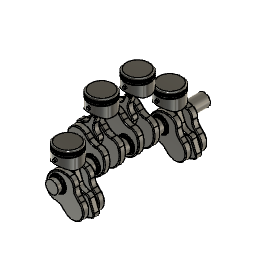
piston sim (v6~recovered) (Autodesk Fusion 360 design; units mm, degrees)
Autodesk Fusion 360 part; units mm, degrees
note: some values were not read from the file. Set by a fixed rule: which face or edge a step refers to.
sketch "Sketch1" plane through (0, 0, 0) normal (0, 1, 0) x (1, 0, 0) in component "piston2"
  line L0 (0, 0) -> (40, 0)
  line L1 (40, 0) -> (40, -55)
  line L2 (40, -55) -> (0, -55)
  line L3 (0, -55) -> (0, 0)
  line L4 (40, -48) -> (36, -48)
  line L5 (36, -48) -> (36, -46)
  line L6 (36, -46) -> (40, -46)
  line L7 (40, -46) -> (40, -48)
  line L8 (40, -44) -> (36, -44)
  line L9 (36, -44) -> (36, -42)
  line L10 (36, -42) -> (40, -42)
  line L11 (40, -42) -> (40, -44)
  line L12 (40, -38) -> (36, -38)
  line L13 (36, -38) -> (36, -36)
  line L14 (36, -36) -> (40, -36)
  line L15 (40, -36) -> (40, -38)
  dimension "d1" = 40
  dimension "d2" = 55
  dimension "d3" = 2
  dimension "d4" = 7
  dimension "d5" = 4
  dimension "d6" = 4
  dimension "d7" = 2
  dimension "d8" = 2
  dimension "d9" = 4
  dimension "d10" = 2
  dimension "d11" = 4
  constraint horizontal L0
  constraint vertical L1
  constraint horizontal L2
  constraint vertical L3
  constraint coincident L0.start L3.end
  constraint horizontal L4
  constraint vertical L5
  constraint horizontal L6
  constraint vertical L7
  constraint coincident L1 L4.start
  constraint horizontal L8
  constraint vertical L9
  constraint horizontal L10
  constraint vertical L11
  constraint coincident L1 L8.start
  constraint horizontal L12
  constraint vertical L13
  constraint horizontal L14
  constraint vertical L15
  constraint coincident L1 L12.start
  measures "d1" distance of L0.start L0.end
  measures "d2" distance of L0.start L2.end
  measures "d3" distance of L4.end L5.end
  measures "d4" distance of L1.end L4.start
  measures "d5" distance of L4.start L4.end
  measures "d6" distance of L8.start L8.end
  measures "d7" distance of L8.end L9.end
  measures "d8" distance of L12.end L13.end
  measures "d9" distance of L12.start L12.end
  measures "d10" distance of L6.end L8.start
  measures "d11" distance of L10.end L12.start
revolve "Revolve1" add sketch "Sketch1" angle 360 about axis through (0, 0, 55) along (0, 0, -1) contours L0 L1 L2 L3 L4 L5 L6 L8 L9 L10 L12 L13 L14 makes body 1 in component "piston2"
fillet "Fillet1" radius 5 1 edges at (-37.2931, -14.4646, 55) on bodies 1 in component "piston2"
sketch "Sketch2" plane through (0, 0, 0) normal (0, 0, -1) x (1, 0, 0) in component "piston2"
  circle A0 centre (0, 0) radius 40
  circle A1 centre (0, 0) radius 35
  dimension "d15" = 70
  constraint coincident A0.centre A1.centre
  measures "d15" diameter of A1
extrude "Extrude1" cut sketch "Sketch2" against normal blind 50 contours A1 bodies 1 in component "piston2"
sketch "Sketch3" plane through (0, 0, 0) normal (0, 1, 0) x (1, 0, 0) in component "piston2"
  line L0 (-40, 0) -> (40, 0)
  line L1 (-40, -36) -> (40, -36)
  line L2 (0, 0) -> (0, -10)
  circle A0 centre (0, -24) radius 5
  arc A1 (-35, 0) -> (35.5, 0) centre (0.25, 56.0937) ccw
  point P0 (-35, 0)
  dimension "d18" = 10
  dimension "d19" = 10
  dimension "d22" = 5
  dimension "d23" = 4.5
  dimension "d24" = 5
  dimension "d25" = 24
  constraint coincident L2.start origin
  constraint perpendicular L0 L2
  constraint coincident L0 A1.end
  constraint coincident P0 A1.start
  measures "d18" distance of L2.start L2.end
  measures "d19" diameter of A0
  measures "d22" distance of L0.start P0
  measures "d23" distance of L0.end A1.end
  measures "d24" distance of L0.start P0
  measures "d25" distance of L2.start A0.centre
extrude "Extrude2" cut sketch "Sketch3" along normal blind 45 and the other way blind 55 bodies 1 in component "piston2"
pattern_linear "00000000-0000-0000-0000-000000000000" [suppressed] in component "pistons"
sketch "Sketch1 (2)" plane through (0, 0, 0) normal (0, 1, 0) x (1, 0, 0) in component "connecting rod"
  circle A0 centre (0, -75) radius 5
  circle A1 centre (0, -75) radius 8.5
  circle A2 centre (0, 50) radius 22.5
  line L0 (8.5, -75) -> (8.5, 0)
  line L1 (0, 50) -> (36, 50)
  line L2 (36, 50) -> (36, 25)
  line L3 (36, 25) -> (33.5, 25)
  arc A3 (33.5, 25) -> (8.5, 0) centre (33.5, 0) ccw
  line L4 (0, 0) -> (0, 50) construction
  line L5 (-8.5, -75) -> (-8.5, 0)
  arc A4 (-8.5, 0) -> (-33.5, 25) centre (-33.5, 0) ccw
  line L6 (-36, 50) -> (-36, 25)
  line L7 (-36, 25) -> (-33.5, 25)
  line L8 (0, 50) -> (-36, 50)
  line L9 (-36, 50) -> (36, 50)
  line L10 (36, 50) -> (36, 86)
  line L11 (36, 86) -> (-36, 86)
  line L12 (-36, 86) -> (-36, 50)
  circle A5 centre (0, -60) radius 4.75
  circle A6 centre (0, -23) radius 4.75
  line L13 (-4.75, -60) -> (-4.75, -23)
  line L14 (4.75, -60) -> (4.75, -23)
  dimension "d34" = 10
  dimension "d35" = 17
  dimension "d36" = 45
  dimension "d37" = 125
  dimension "d39" = 36
  dimension "d40" = 25
  dimension "d41" = 25
  dimension "d42" = 36
  dimension "d47" = 9.5
  dimension "d48" = 15
  dimension "d49" = 15
  dimension "d60" = 37
  dimension "d61" = 9.5
  constraint concentric A0 A1
  constraint coincident A1 L0.start
  constraint tangent A1 L0
  constraint vertical L0
  constraint coincident A2.centre L1.start
  constraint horizontal L1
  constraint perpendicular L1 L2
  constraint perpendicular L0 L3
  constraint tangent L3 A3
  constraint tangent L0 A3
  constraint coincident L4.start origin
  constraint perpendicular L1 L4
  constraint symmetric L0.start L4 L5.start
  constraint symmetric A2.centre L4 L1.start
  constraint symmetric L1.end L4 L6.start
  constraint symmetric L2.end L4 L6.end
  constraint symmetric L3.end L4 A4.end
  constraint symmetric L0.end L4 L5.end
  constraint symmetric A3 L4 A4
  constraint horizontal L9
  constraint vertical L10
  constraint horizontal L11
  constraint vertical L12
  constraint coincident A5 L13.start
  constraint tangent A5 L13
  constraint coincident A6 L13.end
  constraint tangent A6 L13
  constraint vertical L13
  constraint coincident A5 L14.start
  constraint tangent A5 L14
  constraint coincident A6 L14.end
  constraint tangent A6 L14
  measures "d34" diameter of A0
  measures "d35" diameter of A1
  measures "d36" diameter of A2
  measures "d37" distance of A0.centre A2.centre
  measures "d39" distance of A2.centre L1.end
  measures "d40" distance of L1.end L2.end
  measures "d41" radius of A3
  measures "d42" distance of L6.start L11.end
  measures "d47" diameter of A5
  measures "d48" distance of A0.centre A5.centre
  measures "d49" distance of A0.centre A5.centre
  measures "d60" distance of A5.centre A6.centre
  measures "d61" diameter of A6
extrude "Extrude1'" add sketch "Sketch1 (2)" along normal mid plane 20 separate body contours A1 | A1 A2 L0 L1 L2 L3 A3 L5 A4 L6 L7 L8 L9 | A2 L1 L8 L9 L10 L11 L12 makes body 2 in component "connecting rod"
extrude "Extrude2'" add sketch "Sketch1 (2)" along normal mid plane 10 contours A5 | A5 A6 L13 L14 | A6 bodies 2 in component "connecting rod"
fillet "Fillet1'" radius 12.5 4 edges at (36, 0, -25) (36, 0, -86) (-36, 0, -25) (-36, 0, -86) on bodies 2 in component "connecting rod"
fillet "Fillet2" radius 2.5 24 edges at (-8.5, -10, 37.5) (-13.6044, -10, -15.1383) (-33.4478, -10, -28.573) (-36, -10, -54.821) (-32.3388, -10, -82.3388) (0, -10, -86) (32.3388, -10, -82.3388) (36, -10, -54.821) (33.4478, -10, -28.573) (13.6044, -10, -15.1383) (8.5, -10, 37.5) (0, -10, 83.5) (33.4478, 10, -28.573) (36, 10, -54.821) (32.3388, 10, -82.3388) (0, 10, -86) (-32.3388, 10, -82.3388) (-36, 10, -54.821) (-33.4478, 10, -28.573) (-13.6044, 10, -15.1383) (-8.5, 10, 37.5) (0, 10, 83.5) (8.5, 10, 37.5) (13.6044, 10, -15.1383) on bodies 2 in component "connecting rod"
fillet "Fillet3" radius 1.5 16 edges at (4.75, -10, 41.5) (0, -10, 18.25) (-4.75, -10, 41.5) (0, -10, 64.75) (4.75, -5, 41.5) (0, -5, 18.25) (-4.75, -5, 41.5) (0, -5, 64.75) (-4.75, 5, 41.5) (0, 5, 18.25) (4.75, 5, 41.5) (0, 5, 64.75) (4.75, 10, 41.5) (0, 10, 64.75) (-4.75, 10, 41.5) (0, 10, 18.25) on bodies 2 in component "connecting rod"
pattern_linear "00000000-0000-0000-0000-000000000000'" [suppressed] in component "connecting rods"
sketch "Sketch1 (3)" plane through (0, 0, 0) normal (0, 1, 0) x (1, 0, 0) in component "pin"
  circle A0 centre (10, -130) radius 5
  dimension "d76" = 10
  measures "d76" diameter of A0
extrude "Extrude1''" add sketch "Sketch1 (3)" against normal blind 90 separate body makes body 3 in component "pin"
fillet "Fillet1''" radius 1.5 2 edges at (5.3384, -90, 128.1919) (5.3384, 0, 131.8081) on bodies 3 in component "pin"
pattern_linear "00000000-0000-0000-0000-000000000000''" [suppressed] in component "pins"
sketch "Sketch1 (4)" plane through (0, 0, 0) normal (0, 1, 0) x (1, 0, 0) in component "crankshaft"
  circle A0 centre (0, 50) radius 22.5
  circle A1 centre (0, 50) radius 35
  circle A2 centre (0, -14.5) radius 20
  circle A3 centre (0, -14.5) radius 25
  line L0 (-35, 7.5) -> (-55, 7.5)
  arc A4 (-55, 7.5) -> (55, 7.5) centre (0, 7.5) ccw
  line L1 (-35, 50) -> (-35, 7.5)
  line L2 (35, 50) -> (35, 7.5)
  line L3 (35, 7.5) -> (55, 7.5)
  dimension "d85" = 70
  dimension "d87" = 40
  dimension "d88" = 50
  constraint concentric A0 A1
  constraint concentric A2 A3
  constraint horizontal L0
  constraint coincident A1 L1.start
  constraint tangent A1 L1
  constraint perpendicular L0 L1
  constraint coincident A1 L2.start
  constraint tangent A1 L2
  measures "d85" diameter of A1
  measures "d87" diameter of A2
  measures "d88" diameter of A3
extrude "Extrude1'''" add sketch "Sketch1 (4)" against normal blind 20 from surface at -15 separate body contours A0 | A1 | A1 L0 A4 L1 L2 L3 | A2 | A3 makes body 4 in component "crankshaft"
extrude "Extrude2''" add sketch "Sketch1 (4)" against normal blind 20 from surface at -35 contours A2 bodies 4 in component "crankshaft"
extrude "Extrude3" add sketch "Sketch1 (4)" against normal blind 5 from surface at -35 contours A3 bodies 4 in component "crankshaft"
fillet "Fillet1'''" radius 30 2 edges at (35, -25, -7.5) (-35, -25, -7.5) on bodies 4 in component "crankshaft"
fillet "Fillet2'" radius 25 2 edges at (55, -25, -7.5) (-55, -25, -7.5) on bodies 4 in component "crankshaft"
fillet "Fillet3'" radius 2.5 16 edges at (-51.987, -35, -0.6375) (-37.4915, -35, -23.8142) (-35, -35, -42.8921) (0, -35, -85) (35, -35, -42.8921) (37.4915, -35, -23.8142) (51.987, -35, -0.6375) (0, -35, 47.5) (0, -15, 47.5) (-51.987, -15, -0.6375) (-37.4915, -15, -23.8142) (-35, -15, -42.8921) (0, -15, -85) (35, -15, -42.8921) (37.4915, -15, -23.8142) (51.987, -15, -0.6375) on bodies 4 in component "crankshaft"
fillet "Fillet4" radius 1.5 3 edges at (-18.6465, -40, 7.2677) (-23.3082, -40, 5.4596) (-23.3082, -35, 23.5404) on bodies 4 in component "crankshaft"
mirror "Mirror1" about plane through (0, 0, 0) normal (0, 1, 0) of bodies 4 makes body 5 in component "crankshaft"
extrude "Extrude4" add sketch "Sketch1 (4)" along normal mid plane 30 contours A0 bodies 4 5 in component "crankshaft"
pattern_linear "R-Pattern1" count 4 spacing 110 along (0, -1, 0) of bodies 4 makes body 6 at (-26.5501, -125, -3.8431) makes body 7 at (-26.5501, -235, -3.8431) makes body 8 at (-26.5501, -345, -3.8431) in component "crankshaft"
move_body "Move1" bodies 7 6 to x (-1, 0, 0) y (0, 1, 0) z (0, 0, -1) at (0, 0, 29) in component "crankshaft"
combine "Combine1" operation add target body 8 tool bodies 7 6 4 in component "crankshaft"
extrude "Extrude5" add 1 faces at (6.7345, 55, 17.3926) along direction (0, 1, 0) blind 50 on bodies 8 bodies 8 in component "crankshaft"
sketch "Sketch1 (5)" plane through (0, 105, 0) normal (0, 1, 0) x (-1, 0, 0)
  circle A0 centre (0, 14.5) radius 20
  circle A1 centre (0, 14.5) radius 37.5
  dimension "d118" = 75
  constraint concentric A0 A1
  measures "d118" diameter of A1
extrude "Extrude1''''" add sketch "Sketch1 (5)" against normal blind 20 separate body makes body 9 in component "Component'"
sketch "Sketch2 (2)" plane through (0, 0, 235) normal (0, 0, 1) x (-1, 0, 0)
  circle A0 centre (0, 213.2476) radius 35
  line L0 (211.5692, -160.9153) -> (-250, -160.9153)
  line L1 (-250, -160.9153) -> (-250, 450)
  line L2 (-250, 450) -> (211.5692, 450)
  line L3 (211.5692, 450) -> (211.5692, -160.9153)
  circle A1 centre (0, 321.7476) radius 40
  circle A2 centre (0, 213.2476) radius 40
  circle A3 centre (0, 97.2476) radius 40
  circle A4 centre (0, -6.7524) radius 40
  constraint horizontal L0
  constraint vertical L1
  constraint horizontal L2
  constraint vertical L3
extrude "Extrude1'''''" add sketch "Sketch2 (2)" along normal blind 25 separate body contours L0 L1 L2 L3 makes body 10 in component "Component''"
component "pistons" placed x (1, 0, 0) y (0, 1, 0) z (0, 0, 1) at (0, 0, 0)
component "Component" placed x (1, 0, 0) y (0, 1, 0) z (0, 0, 1) at (0, 0, 0)
component "connecting rods" placed x (1, 0, 0) y (0, 1, 0) z (0, 0, 1) at (0, 0, 0)
component "pins" placed x (1, 0, 0) y (0, 1, 0) z (0, 0, 1) at (0, 0, 0)
component "crankshaft" placed x (-1, 0, 0) y (0, 1, 0) z (0, 0, -1) at (0, 11.75, 29)
component "Component'" placed x (1, 0, 0) y (0, 1, 0) z (0, 0, 1) at (0, 0, 0)
component "Component''" placed x (1, 0, 0) y (0, 1, 0) z (0, 0, 1) at (0, 0, 0)
component "piston2" placed x (1, 0, 0) y (0, 1, 0) z (0, 0, 1) at (0, 6.7524, 180) in component "pistons"
component "piston2" placed x (1, 0, 0) y (0, 1, 0) z (0, 0, 1) at (0, -97.2476, 51) in component "pistons"
component "piston2" placed x (1, 0, 0) y (0, 1, 0) z (0, 0, 1) at (0, -213.2476, 51) in component "pistons"
component "piston2" placed x (1, 0, 0) y (0, 1, 0) z (0, 0, 1) at (0, -321.7476, 180) in component "pistons"
component "connecting rod" placed x (1, 0, 0) y (0, 1, 0) z (0, 0, 1) at (0, 11.75, 129) in component "connecting rods"
component "connecting rod" placed x (1, 0, 0) y (0, 1, 0) z (0, 0, 1) at (0, -97.25, 0) in component "connecting rods"
component "connecting rod" placed x (1, 0, 0) y (0, 1, 0) z (0, 0, 1) at (0, -208.25, 0) in component "connecting rods"
component "connecting rod" placed x (1, 0, 0) y (0, 1, 0) z (0, 0, 1) at (0, -317.25, 129) in component "connecting rods"
component "pin" placed x (1, 0, 0) y (0, 1, 0) z (0, 0, 1) at (-10, 51.75, 74) in component "pins"
component "pin" placed x (1, 0, 0) y (0, 1, 0) z (0, 0, 1) at (-10, -52.25, -55) in component "pins"
component "pin" placed x (1, 0, 0) y (0, 1, 0) z (0, 0, 1) at (-10, -168.25, -55) in component "pins"
component "pin" placed x (1, 0, 0) y (0, 1, 0) z (0, 0, 1) at (-10, -277.25, 74) in component "pins"
